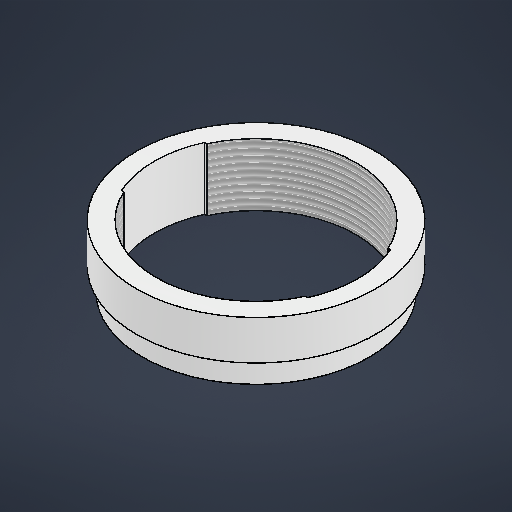
# Autodesk Inventor part: Bottom Nut
Saved by Autodesk Inventor 2026 (Build 300175050, 175E)
## iProperties
Created: 2025-06-28
Part Number: Bottom Nut
Material: ABS Plastic
Document SubType Name: Modeling
Designer: Joshua Eah
Density: 1.06 g/cm^3
Appearance: Smooth - White
Author: Joshua Eah
Autodesk Inventor part; units mm, degrees
ref_plane "YZ Plane" through (0, 0, 0) normal (1, 0, 0) x (0, 1, 0)
ref_plane "XZ Plane" through (0, 0, 0) normal (0, 1, 0) x (-1, 0, 0)
ref_plane "XY Plane" through (0, 0, 0) normal (0, 0, 1) x (1, 0, 0)
sketch "Sketch1" plane through (0, 0, 0) normal (0, 1, 0) x (-1, 0, 0)
  circle A0 centre (0, 0) radius 14.375
  circle A1 centre (0, 0) radius 12
  circle A2 centre (0, 0) radius 13.625
  circle A3 centre (0, 0) radius 12.25
  line L0 (12.25, -5) -> (-12.25, -5)
  line L1 (-12.25, -5) -> (-12.25, 5)
  line L2 (-12.25, 5) -> (12.25, 5)
  line L3 (12.25, 5) -> (12.25, -5)
  line L4 (12.25, -5) -> (-12.25, 5) construction
  line L5 (-12.25, -5) -> (12.25, 5) construction
  point P0 (-10.9087, 5)
  point P1 (-11.1831, 5)
  point P2 (-11.1831, -5)
  point P3 (-10.9087, -5)
  point P4 (11.1831, 5)
  point P5 (10.9087, 5)
  point P6 (10.9087, -5)
  point P7 (11.1831, -5)
  dimension "d0" = 28.75
  dimension "d1" = 24
  dimension "d4" = 27.25
  dimension "d9" = 24.5
  dimension "d10" = 10
  constraints: 12 end point, 4 centre point, 4 coincident, 2 midpoint, 2 parallel, 1 horizontal, 1 perpendicular, 1 tangent
  measures "d0" diameter of A0
  measures "d1" diameter of A1
  measures "d4" diameter of A2
  measures "d9" diameter of A3
  measures "d10" distance of L0.end L1.end
extrude "Extrusion1" add sketch "Sketch1" along normal blind 7.5 contours A0 | A1 L2 A3 L0 | A1 L2 A3 | L0 A3 A1 | A1 L0 A3 L2 | L2 L3 A3 | A3 L3 L0 | A3 L1 L2 | L0 L1 A3 | A2
extrude "Extrusion2" cut sketch "Sketch1" along normal blind 2.75 contours A0
thread "Thread1" size "M24x0.75" class "6H" standard "ANSI Metric M Profile" full length
extrude "Extrusion3" cut sketch "Sketch1" along normal through all contours A1 L2 A3 L0 | A1 L0 A3 L2
body "Solid1"
